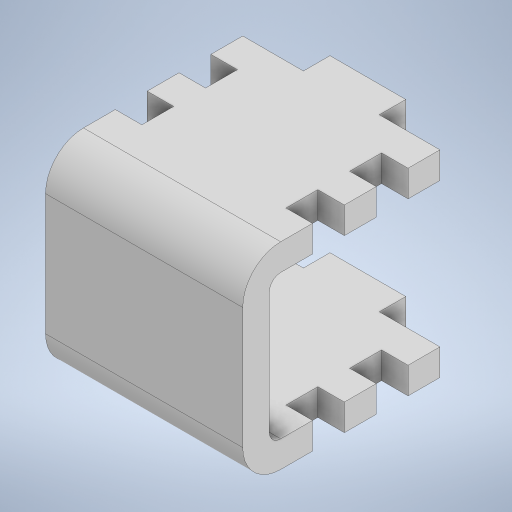
# Autodesk Inventor part: Spodnji del - Upognjen les
Saved by Autodesk Inventor 2023 (Build 270158000, 158)
## iProperties
Created: 2022-12-16
Part Number: Spodnji del - Upognjen les
Material: Generic
Document SubType Name: Modeling
Designer: David Zindović
Density: 1 g/cm^3
Appearance: Default
Author: David Zindović
Autodesk Inventor part; units mm, degrees
ref_plane "YZ Plane" through (0, 0, 0) normal (1, 0, 0) x (0, 1, 0)
ref_plane "XZ Plane" through (0, 0, 0) normal (0, 1, 0) x (-1, 0, 0)
sketch "Sketch1" plane through (0, 0, 0) normal (1, 0, 0) x (0, 1, 0)
  line L0 (13, 8) -> (13, -13)
  line L1 (5, -13) -> (0, -13)
  line L2 (0, -16.5) -> (5, -16.5)
  line L3 (5, -16.5) -> (5, -13)
  line L4 (0, 7.0803) -> (-6.4131, 0.6672)
  line L5 (-7.0965, 1.3506) -> (-0.3417, 8.1054)
  line L6 (-7.9849, 0.4622) -> (-7.0965, 1.3506) construction
  spline S0 degree 3 poles (-8.4777, -1.9692) (-8.4777, -0.714) (-7.9849, 0.4622) (-7.0965, 1.3506) knots 7 7 7 7 8 8 8 8
  line L7 (-8.4777, -1.9692) -> (-8.4777, -0.714) construction
  line L8 (-8.4777, -0.714) -> (-7.9849, 0.4622) construction
  line L9 (-6.4131, 0.6672) -> (-7.1181, -0.0378) construction
  spline S1 degree 3 poles (-6.4131, 0.6672) (-7.1181, -0.0378) (-7.5065, -0.9729) (-7.5065, -1.9692) (-7.5065, -2.9656) (-7.1217, -3.9007) (-6.4167, -4.6021) knots 2 2 2 2 3 3 3 4 4 4 4
  line L10 (-7.1181, -0.0378) -> (-7.5065, -0.9729) construction
  line L11 (-7.5065, -0.9729) -> (-7.5065, -1.9692) construction
  line L12 (-7.5065, -1.9692) -> (-7.5065, -2.9656) construction
  line L13 (-7.5065, -2.9656) -> (-7.1217, -3.9007) construction
  line L14 (-7.1217, -3.9007) -> (-6.4167, -4.6021) construction
  line L15 (-8.4813, -3.2245) -> (-8.4777, -1.9692) construction
  spline S2 degree 3 poles (-7.1037, -5.2927) (-7.9921, -4.4043) (-8.4813, -3.2245) (-8.4777, -1.9692) knots 6 6 6 6 7 7 7 7
  line L16 (-7.1037, -5.2927) -> (-7.9921, -4.4043) construction
  line L17 (-7.9921, -4.4043) -> (-8.4813, -3.2245) construction
  line L18 (-1.1474, -4.5985) -> (-0.3345, -3.7856)
  line L19 (-1.8524, -5.3035) -> (-1.1474, -4.5985) construction
  spline S3 degree 3 poles (-6.4167, -4.6021) (-5.7153, -5.3035) (-4.7802, -5.6919) (-3.7874, -5.6919) (-2.7911, -5.6919) (-1.8524, -5.3035) (-1.1474, -4.5985) knots 4 4 4 4 5 5 5 6 6 6 6
  line L20 (-6.4167, -4.6021) -> (-5.7153, -5.3035) construction
  line L21 (-5.7153, -5.3035) -> (-4.7802, -5.6919) construction
  line L22 (-4.7802, -5.6919) -> (-3.7874, -5.6919) construction
  line L23 (-3.7874, -5.6919) -> (-2.7911, -5.6919) construction
  line L24 (-2.7911, -5.6919) -> (-1.8524, -5.3035) construction
  line L25 (-0.4604, -5.2855) -> (-1.3488, -6.1739) construction
  spline S4 degree 3 poles (-0.4604, -5.2855) (-1.3488, -6.1739) (-2.5321, -6.6667) (-3.7874, -6.6667) (-5.0391, -6.6667) (-6.2189, -6.1775) (-7.1037, -5.2927) knots 4 4 4 4 5 5 5 6 6 6 6
  line L26 (-1.3488, -6.1739) -> (-2.5321, -6.6667) construction
  line L27 (-2.5321, -6.6667) -> (-3.7874, -6.6667) construction
  line L28 (-3.7874, -6.6667) -> (-5.0391, -6.6667) construction
  line L29 (-5.0391, -6.6667) -> (-6.2189, -6.1775) construction
  line L30 (-6.2189, -6.1775) -> (-7.1037, -5.2927) construction
  line L31 (2.5429, -6.6559) -> (1.3632, -6.1667) construction
  spline S5 degree 3 poles (7.1181, -5.2819) (6.2297, -6.1703) (5.0535, -6.6559) (3.7982, -6.6559) (2.5429, -6.6559) (1.3632, -6.1667) (0.4748, -5.2783) knots 0 0 0 0 1 1 1 2 2 2 2
  line L32 (7.1181, -5.2819) -> (6.2297, -6.1703) construction
  line L33 (6.2297, -6.1703) -> (5.0535, -6.6559) construction
  line L34 (5.0535, -6.6559) -> (3.7982, -6.6559) construction
  line L35 (3.7982, -6.6559) -> (2.5429, -6.6559) construction
  line L36 (1.3632, -6.1667) -> (0.4748, -5.2783) construction
  spline S6 degree 3 poles (-0.3345, -3.7856) (-0.1439, -3.595) (0.1619, -3.595) (0.3525, -3.7856) knots 7 7 7 7 8 8 8 8
  line L37 (-0.1439, -3.595) -> (0.1619, -3.595) construction
  line L38 (-0.3345, -3.7856) -> (-0.1439, -3.595) construction
  line L39 (0.1619, -3.595) -> (0.3525, -3.7856) construction
  line L40 (0.0108, -4.8143) -> (-0.4604, -5.2855)
  line L41 (0.4748, -5.2783) -> (0.0108, -4.8143)
  line L42 (6.4275, 0.678) -> (0, 7.0803)
  line L43 (-0.3417, 8.1054) -> (-0.2482, 8.1989) construction
  spline S7 degree 3 poles (-0.3417, 8.1054) (-0.2482, 8.1989) (-0.1223, 8.2493) (0, 8.2493) (0.1223, 8.2493) (0.2482, 8.2025) (0.3417, 8.109) knots 9 9 9 9 10 10 10 11 11 11 11
  line L44 (-0.2482, 8.1989) -> (-0.1223, 8.2493) construction
  line L45 (-0.1223, 8.2493) -> (0, 8.2493) construction
  line L46 (0, 8.2493) -> (0.1223, 8.2493) construction
  line L47 (0.1223, 8.2493) -> (0.2482, 8.2025) construction
  line L48 (0.2482, 8.2025) -> (0.3417, 8.109) construction
  line L49 (0.3417, 8.109) -> (7.1109, 1.365)
  line L50 (0.3525, -3.7856) -> (1.1582, -4.5913)
  spline S8 degree 3 poles (1.1582, -4.5913) (1.8631, -5.2963) (2.8019, -5.6847) (3.7946, -5.6847) (4.7873, -5.6847) (5.7225, -5.2963) (6.4275, -4.5949) knots 9 9 9 9 10 10 10 11 11 11 11
  line L51 (1.1582, -4.5913) -> (1.8631, -5.2963) construction
  line L52 (1.8631, -5.2963) -> (2.8019, -5.6847) construction
  line L53 (2.8019, -5.6847) -> (3.7946, -5.6847) construction
  line L54 (3.7946, -5.6847) -> (4.7873, -5.6847) construction
  line L55 (4.7873, -5.6847) -> (5.7225, -5.2963) construction
  line L56 (5.7225, -5.2963) -> (6.4275, -4.5949) construction
  line L57 (6.4275, -4.5949) -> (7.1325, -3.8899) construction
  spline S9 degree 3 poles (6.4275, -4.5949) (7.1325, -3.8899) (7.5173, -2.9548) (7.5173, -1.9584) knots 11 11 11 11 12 12 12 12
  line L58 (7.1325, -3.8899) -> (7.5173, -2.9548) construction
  line L59 (7.5173, -2.9548) -> (7.5173, -1.9584) construction
  line L60 (8.0065, -4.3935) -> (7.1181, -5.2819) construction
  spline S10 degree 3 poles (8.4885, -1.9584) (8.4921, -3.2137) (8.0065, -4.3935) (7.1181, -5.2819) knots 13 13 13 13 14 14 14 14
  line L61 (8.4885, -1.9584) -> (8.4921, -3.2137) construction
  line L62 (8.4921, -3.2137) -> (8.0065, -4.3935) construction
  line L63 (7.5173, -1.9584) -> (7.5209, -0.9621) construction
  spline S11 degree 3 poles (7.5173, -1.9584) (7.5209, -0.9621) (7.1325, -0.027) (6.4275, 0.678) knots 12 12 12 12 13 13 13 13
  line L64 (7.5209, -0.9621) -> (7.1325, -0.027) construction
  line L65 (7.1325, -0.027) -> (6.4275, 0.678) construction
  line L66 (8.4885, -0.7032) -> (8.4885, -1.9584) construction
  spline S12 degree 3 poles (7.1109, 1.365) (7.9993, 0.4766) (8.4885, -0.7032) (8.4885, -1.9584) knots 12 12 12 12 13 13 13 13
  line L67 (7.1109, 1.365) -> (7.9993, 0.4766) construction
  line L68 (7.9993, 0.4766) -> (8.4885, -0.7032) construction
  arc A0 (13, 8) -> (8, 13) centre (8, 8) ccw
  line L69 (0, -16.5) -> (0, -13)
  line L70 (13, -13) -> (0, -13)
  line L71 (8, 13) -> (0, 13)
  line L72 (-8, 13) -> (0, 13)
  arc A1 (-8, 13) -> (-13, 8) centre (-8, 8) ccw
  line L73 (-5, -13) -> (0, -13)
  line L74 (-5, -16.5) -> (-5, -13)
  line L75 (0, -16.5) -> (-5, -16.5)
  line L76 (-13, -13) -> (0, -13)
  line L77 (-13, 8) -> (-13, -13)
  line L78 (13, -4.6) -> (16.5, -4.6)
  line L79 (16.5, -4.6) -> (16.5, -8.8)
  line L80 (16.5, -8.8) -> (13, -8.8)
  line L81 (13, -8.8) -> (13, -4.6)
  line L82 (16.5, -0.4) -> (13, -0.4)
  line L83 (16.5, 3.8) -> (16.5, -0.4)
  line L84 (13, 3.8) -> (16.5, 3.8)
  line L85 (-16.5, 3.8) -> (-16.5, -0.4)
  line L86 (-13, 3.8) -> (-16.5, 3.8)
  line L87 (-16.5, -0.4) -> (-13, -0.4)
  line L88 (-13, -4.6) -> (-16.5, -4.6)
  line L89 (-16.5, -8.8) -> (-13, -8.8)
  line L90 (-16.5, -4.6) -> (-16.5, -8.8)
  line L91 (9.5, -9.5) -> (9.5, 8)
  arc A2 (9.5, 8) -> (8, 9.5) centre (8, 8) ccw
  line L92 (8, 9.5) -> (0, 9.5)
  line L93 (0, 9.5) -> (-8, 9.5)
  arc A3 (-8, 9.5) -> (-9.5, 8) centre (-8, 8) ccw
  line L94 (-9.5, 8) -> (-9.5, -9.5)
  line L95 (-9.5, -9.5) -> (0, -9.5)
  line L96 (0, -9.5) -> (9.5, -9.5)
  line L97 (9.5, -9.5) -> (9.5, -13)
  line L98 (-9.5, -9.5) -> (-9.5, -13)
  line L99 (13, -8.8) -> (9.5, -8.8)
  line L100 (9.5, -8.8) -> (9.5, -4.6)
  line L101 (9.5, -4.6) -> (13, -4.6)
  line L102 (13, -4.6) -> (13, -8.8)
  line L103 (13, -0.4) -> (9.5, -0.4)
  line L104 (9.5, -0.4) -> (9.5, 3.8)
  line L105 (9.5, 3.8) -> (13, 3.8)
  line L106 (13, 3.8) -> (13, -0.4)
  line L107 (-13, 3.8) -> (-9.5, 3.8)
  line L108 (-9.5, 3.8) -> (-9.5, -0.4)
  line L109 (-9.5, -0.4) -> (-13, -0.4)
  line L110 (-13, -0.4) -> (-13, 3.8)
  line L111 (-13, -4.6) -> (-9.5, -4.6)
  line L112 (-9.5, -4.6) -> (-9.5, -8.8)
  line L113 (-9.5, -8.8) -> (-13, -8.8)
  line L114 (-13, -8.8) -> (-13, -4.6)
  line L115 (0.3, 6.198) -> (-0.3, 6.198)
  line L116 (-0.3, 6.198) -> (-0.3, 9.1381)
  line L117 (-0.3, 9.1381) -> (0.3, 9.1381)
  line L118 (0.3, 9.1381) -> (0.3, 6.198)
  line L119 (-8.0638, -4.3092) -> (-5.5177, -2.8392)
  line L120 (-7.7638, -4.8289) -> (-8.0638, -4.3092)
  line L121 (-5.2177, -3.3588) -> (-7.7638, -4.8289)
  line L122 (-5.5177, -2.8392) -> (-5.2177, -3.3588)
  line L123 (7.7638, -4.8289) -> (5.2177, -3.3588)
  line L124 (8.0638, -4.3092) -> (7.7638, -4.8289)
  line L125 (5.5177, -2.8392) -> (8.0638, -4.3092)
  line L126 (5.2177, -3.3588) -> (5.5177, -2.8392)
  point P0 (0.3, 11.1366)
  point P1 (0.4643, 11.0177)
  point P2 (9.6684, 1.8477)
  point P3 (11.5332, -2.6643)
  point P4 (10.7976, -5.6567)
  point P5 (9.6497, -4.9939)
  point P6 (10.2137, -2.6609)
  point P7 (8.7384, 0.9158)
  point P8 (0.5, 9.122)
  point P9 (10.2596, -6.5007)
  point P10 (9.6713, -7.1765)
  point P11 (0.6451, -7.1716)
  point P12 (0.0147, -6.5412)
  point P13 (-0.6255, -7.1814)
  point P14 (-9.6517, -7.1911)
  point P15 (-10.2539, -6.4975)
  point P16 (-9.2214, -5.6704)
  point P17 (-8.7205, -6.2507)
  point P18 (-1.5589, -6.248)
  point P19 (-0.4542, -5.1432)
  point P20 (0.4789, -5.1435)
  point P21 (1.5736, -6.2382)
  point P22 (8.733, -6.2431)
  point P23 (9.102, -5.8324)
  point P24 (-0.3, 11.1333)
  point P25 (-0.5, 9.12)
  point P26 (-8.7136, 0.9064)
  point P27 (-9.5487, -5.1665)
  point P28 (-10.7898, -5.6522)
  point P29 (-11.5186, -2.6721)
  point P30 (-9.642, 1.8351)
  point P31 (-0.4643, 11.0128)
  point P32 (8.733, 0.9212)
  point P33 (11.5332, -2.6609)
  point P34 (9.6615, 1.8546)
  point P35 (0.5, 10.9821)
  point P36 (-0.4545, -5.1435)
  point P37 (-8.7183, -6.2528)
  point P38 (-9.0983, -5.8302)
  point P39 (-9.6438, -4.9905)
  point P40 (-11.5186, -2.6756)
  point P41 (-8.7134, 0.9066)
  point P42 (-0.5, 10.977)
  point P43 (0, 0)
  point P44 (13, 13)
  point P45 (-13, 0)
  point P46 (0, 6.5628)
  point P47 (-13, 13)
  point P48 (-5, -14.75)
  point P49 (7.1159, 1.3599)
  point P50 (8.4885, -1.9609)
  point P51 (6.4315, 0.674)
  point P52 (7.1181, -5.2819)
  point P53 (-6.4183, -4.6005)
  point P54 (-0.3345, -3.7856)
  point P55 (1.1582, -4.5913)
  point P56 (-6.4131, 0.6672)
  point P57 (-8.4777, -1.9667)
  point P58 (-0.3417, 8.1054)
  point P59 (8.733, 0.9212)
  point P60 (11.5332, -2.6609)
  point P61 (9.6615, 1.8546)
  point P62 (-0.4545, -5.1435)
  point P63 (-8.7183, -6.2528)
  point P64 (-11.5186, -2.6756)
  point P65 (-8.7134, 0.9066)
  point P66 (0, 6.198)
  point P67 (-5.3677, -3.099)
  point P68 (5.3677, -3.099)
  point P69 (0.3, 8.1463)
  point P70 (7.1109, 1.365)
  point P71 (7.9147, -4.2232)
  point P72 (7.0703, -3.7356)
  point P73 (0.3, 6.7815)
  point P74 (7.5919, -4.7296)
  point P75 (-7.5876, -4.7271)
  point P76 (-6.7441, -4.2401)
  point P77 (-0.3345, -3.7856)
  point P78 (6.7417, -4.2387)
  point P79 (-0.3, 8.1429)
  point P80 (-0.3, 6.7803)
  point P81 (-7.0683, -3.7345)
  point P82 (-7.9091, -4.2199)
  point P83 (-8.4777, -1.9692)
  dimension "d50" = 26
  dimension "d51" = 5
  dimension "d52" = 10
  dimension "d53" = 13
  dimension "d54" = 4.2
  dimension "d55" = 3.5
  dimension "d56" = 4.2
  dimension "d57" = 8.4
  dimension "d58" = 3.5
  dimension "d59" = 0.6
  dimension "d60" = 360
  constraints: 140 end point, 15 symmetric about line, 13 parallel, 13 point on line, 9 horizontal, 9 perpendicular, 8 point on circle, 4 centre point, 3 vertical alignment, 2 midpoint, 1 horizontal alignment, 1 tangent, 1 vertical, 82 other
  measures "d50" distance of point (13, 13) L0.end
  measures "d51" radius of A0
  measures "d52" distance from line of point (-5, -14.75) L3
  measures "d53" distance of L0.end L1.end
  measures "d54" distance of L78.end L79.end
  measures "d55" distance between parallel lines of L0 L79
  measures "d56" distance between parallel lines of L70 L80
  measures "d57" distance of L79.end L82.start
  measures "d58" distance between parallel lines of L0 L91
  measures "d59" distance of L115.start L115.end
extrude "Extrusion1" add sketch "Sketch1" along normal mid plane 26 contours L0 L105 L91 A2 L92 L93 A3 L94 L107 L77 A1 L72 L71 A0 | L0 L103 L91 L105 | L0 L101 L91 L103 | L0 L99 L91 L101 | L0 L70 L97 L91 L99 | L107 L94 L109 L77 | L109 L94 L111 L77 | L111 L94 L113 L77 | L98 L76 L77 L113 L94
sketch "Sketch4" plane through (13, 0, 0) normal (1, 0, 0) x (0, 0, -1)
  line L0 (13, 8) -> (13, -13)
  line L1 (13, -4.6) -> (16.5, -4.6)
  line L2 (16.5, -4.6) -> (16.5, -8.8)
  line L3 (16.5, -8.8) -> (13, -8.8)
  line L4 (16.5, -0.4) -> (13, -0.4)
  line L5 (16.5, 3.8) -> (16.5, -0.4)
  line L6 (13, 3.8) -> (16.5, 3.8)
  line L7 (-0.3, 9.1381) -> (0.3, 9.1381)
  line L8 (-8, 9.5) -> (13, 9.5) projected
  line L9 (8.8, 13.0373) -> (4.6, 13.0373)
  line L10 (4.6, 13.0373) -> (4.6, 9.5)
  line L11 (4.6, 9.5) -> (8.8, 9.5)
  line L12 (8.8, 9.5) -> (8.8, 13.0373)
  line L13 (13, 9.5) -> (13, 13) projected
  line L14 (-3.8, 13.0373) -> (-3.8, 9.5)
  line L15 (0.4, 13.0373) -> (-3.8, 13.0373)
  line L16 (0.4, 9.5) -> (0.4, 13.0373)
  line L17 (-3.8, 9.5) -> (0.4, 9.5)
  line L18 (0, 0) -> (1.8362, 0)
  line L19 (-8, -9.5) -> (13, -9.5)
  line L20 (8.8, -13.0373) -> (4.6, -13.0373)
  line L21 (4.6, -13.0373) -> (4.6, -9.5)
  line L22 (8.8, -9.5) -> (8.8, -13.0373)
  line L23 (-3.8, -13.0373) -> (-3.8, -9.5)
  line L24 (0.4, -13.0373) -> (-3.8, -13.0373)
  line L25 (0.4, -9.5) -> (0.4, -13.0373)
  line L26 (-3.8, -9.5) -> (0.4, -9.5)
  point P0 (0.3417, 8.109)
  point P1 (7.1159, 1.3599)
  point P2 (8.4885, -1.9609)
  point P3 (7.5173, -1.9584)
  point P4 (6.4315, 0.674)
  point P5 (7.1181, -5.2819)
  point P6 (0.4748, -5.2783)
  point P7 (0.0108, -4.8143)
  point P8 (-0.4604, -5.2855)
  point P9 (-7.1037, -5.2927)
  point P10 (-6.4183, -4.6005)
  point P11 (-1.1474, -4.5985)
  point P12 (-0.3345, -3.7856)
  point P13 (0.3525, -3.7856)
  point P14 (1.1582, -4.5913)
  point P15 (6.4275, -4.5949)
  point P16 (-6.4131, 0.6672)
  point P17 (-8.4777, -1.9667)
  point P18 (-7.0965, 1.3506)
  point P19 (-0.3417, 8.1054)
  point P20 (8.733, 0.9212)
  point P21 (11.5332, -2.6609)
  point P22 (9.6615, 1.8546)
  point P23 (-0.4545, -5.1435)
  point P24 (-8.7183, -6.2528)
  point P25 (-11.5186, -2.6756)
  point P26 (-8.7134, 0.9066)
  point P27 (-13, -8.8)
  point P28 (-13, -4.6)
  point P29 (-13, -0.4)
  point P30 (-13, 3.8)
  point P31 (0.3, 8.1463)
  point P32 (7.1109, 1.365)
  point P33 (8.4885, -1.9584)
  point P34 (7.9147, -4.2232)
  point P35 (7.0703, -3.7356)
  point P36 (6.4275, 0.678)
  point P37 (0.3, 6.7815)
  point P38 (7.5919, -4.7296)
  point P39 (-7.5876, -4.7271)
  point P40 (-6.7441, -4.2401)
  point P41 (-6.4167, -4.6021)
  point P42 (-0.3345, -3.7856)
  point P43 (6.7417, -4.2387)
  point P44 (-9.5, 3.8)
  point P45 (-13, 3.8)
  point P46 (-13, -0.4)
  point P47 (-9.5, -4.6)
  point P48 (-13, -4.6)
  point P49 (-13, -8.8)
  point P50 (9.5, -8.8)
  point P51 (9.5, -0.4)
  point P52 (-0.3, 8.1429)
  point P53 (-0.3, 6.7803)
  point P54 (-7.0683, -3.7345)
  point P55 (-7.9091, -4.2199)
  point P56 (-8.4777, -1.9692)
  dimension "d75" = 8.4
  dimension "d80" = 4.2
  dimension "d81" = 4.2
  dimension "d84" = 8.4
  constraints: 50 end point, 10 symmetric about line, 4 horizontal, 3 parallel, 3 point on line, 2 perpendicular, 1 vertical, 15 other
  measures "d75" distance of L2.end L4.start
  measures "d80" distance of L11.end L10.end
  measures "d81" distance between parallel lines of L13 L12
  measures "d84" distance of L9.end L14.start
extrude "Extrusion4" cut sketch "Sketch4" against normal blind 3.5 contours L25 L24 L23 L19 | L22 L20 L21 L19 | L14 L15 L16 L8 | L10 L9 L12 L8
mirror "Mirror3" about plane through (0, 0, 0) normal (1, 0, 0) of "Extrusion4"
sketch "Sketch5" plane through (-13, 13, 8) normal (0, 1, 0) x (1, 0, 0)
  line L0 (0, 21) -> (26, 21) projected
  line L1 (8, 21) -> (18, 21)
  line L2 (18, 21) -> (18, 24.5)
  line L3 (18, 24.5) -> (8, 24.5)
  line L4 (8, 24.5) -> (8, 21)
  point P0 (13, 8)
  point P1 (13, 24.5)
  dimension "d91" = 10
  dimension "d92" = 3.5
  constraints: 8 end point, 2 parallel, 1 horizontal, 1 midpoint, 1 perpendicular, 1 point on line, 1 vertical alignment
  measures "d91" distance of L2.end L3.end
  measures "d92" distance of L1.end L2.end
extrude "Extrusion5" add sketch "Sketch5" against normal up to surface (3.5 mm away)
ref_plane "Work Plane2" through (13, 0, 9.5) normal (0, -1, 0) x (1, 0, 0)
mirror "Mirror4" about plane through (13, 0, 9.5) normal (0, -1, 0) of "Extrusion5"
equation "\"d56\" = d54"
equation "\"d57\" = 2 * d54"
equation "\"d75\" = 2 * d72"
equation "\"d81\" = d80"
equation "\"d84\" = 2 * d80"
equation "\"d72\" = 4.2"
body "Solid1"
